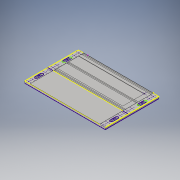
# Autodesk Inventor part: Fixture Base
Saved by Autodesk Inventor 2016 (Build 200138000, 138)
## iProperties
Created: 2016-04-07
Part Number: Fixture Base
Material: Generic
Document SubType Name: Modeling
Designer: Sam Clay
Density: 1 g/cm^3
Appearance: Default
Author: Sam Clay
Autodesk Inventor part; units mm, degrees
ref_plane "YZ Plane" through (0, 0, 0) normal (1, 0, 0) x (0, 1, 0)
ref_plane "XZ Plane" through (0, 0, 0) normal (0, 1, 0) x (-1, 0, 0)
ref_plane "XY Plane" through (0, 0, 0) normal (0, 0, 1) x (1, 0, 0)
sketch "Base Sketch" plane through (0, 0, 0) normal (0, 1, 0) x (-1, 0, 0)
  line L0 (0, 0) -> (660.4, 0)
  line L1 (660.4, 0) -> (660.4, 254)
  line L2 (660.4, 508) -> (0, 508)
  line L3 (0, 508) -> (0, 0)
  line L4 (0, 508) -> (-50.8, 508)
  line L5 (-50.8, 508) -> (-50.8, 254)
  line L6 (-50.8, 0) -> (0, 0)
  line L7 (0, 0) -> (0, 254)
  line L8 (660.4, 508) -> (711.2, 508)
  line L9 (711.2, 508) -> (711.2, 254)
  line L10 (711.2, 0) -> (660.4, 0)
  line L11 (660.4, 0) -> (660.4, 508)
  line L12 (711.2, 254) -> (-50.8, 254)
  line L13 (660.4, 254) -> (660.4, 508)
  line L14 (711.2, 254) -> (711.2, 0)
  line L15 (0, 254) -> (0, 508)
  line L16 (-50.8, 254) -> (-50.8, 0)
  dimension "d0" = 660.4
  dimension "d1" = 508
  dimension "d87" = 50.8
  dimension "d88" = 50.8
  dimension "d118" = 254
  constraints: 34 end point, 11 parallel, 8 perpendicular, 3 horizontal, 3 point on line
  measures "d0" distance of L2.end L2.start
  measures "d1" distance of L2.start L0.end
  measures "d87" distance of L6.end L6.start
  measures "d88" distance of L10.start L10.end
  measures "d118" distance between parallel lines of L0 L12
extrude "Base" add sketch "Base Sketch" along normal blind 19.05 contours L3 L12 L1 L0 | L3 L2 L11 L12
sketch "Tracks Sketch" plane through (0, 19.05, 0) normal (0, 1, 0) x (1, 0, 0)
  line L0 (0, 0) -> (-660.4, 0) projected
  line L1 (-660.4, 0) -> (-660.4, -508) projected
  line L2 (0, 0) -> (-660.4, 0)
  line L3 (-660.4, 0) -> (-660.4, -22.987)
  line L4 (-660.4, -22.987) -> (0, -22.987)
  line L5 (0, -22.987) -> (0, 0)
  line L6 (0, 0) -> (-38.1, 0)
  line L7 (-38.1, 0) -> (-38.1, -251.587)
  line L8 (-38.1, -251.587) -> (0, -251.587)
  line L9 (0, -251.587) -> (0, 0)
  line L10 (-38.1, -284.099) -> (-660.4, -284.099)
  line L11 (-660.4, -284.099) -> (-660.4, -264.287)
  line L12 (-660.4, -264.287) -> (-38.1, -264.287)
  line L13 (-38.1, -264.287) -> (-38.1, -284.099)
  line L14 (0, -48.387) -> (-660.4, -48.387)
  line L15 (-660.4, -48.387) -> (-660.4, -35.687)
  line L16 (-660.4, -35.687) -> (0, -35.687)
  line L17 (0, -35.687) -> (0, -48.387)
  line L18 (-38.1, -42.217) -> (-31.93, -48.387)
  line L19 (-38.1, -42.217) -> (-46.8257, -42.217) construction
  circle A0 centre (-40.4921, -50.7791) radius 8.89
  line L20 (-660.4, -3.175) -> (0, -3.175)
  line L21 (0, -508) -> (0, 0) projected
  line L22 (-38.1, -251.587) -> (-660.4, -251.587)
  line L23 (-660.4, -290.449) -> (0, -290.449)
  line L24 (-38.1, -284.099) -> (0, -284.099)
  line L25 (-38.1, -264.287) -> (0, -264.287)
  line L26 (-660.4, -309.499) -> (0, -309.499)
  line L27 (-660.4, -488.95) -> (0, -488.95)
  line L28 (-660.4, -508) -> (0, -508) projected
  line L29 (-44.45, -309.499) -> (-44.45, -488.95)
  line L30 (-615.95, -309.499) -> (-615.95, -488.95)
  line L31 (-660.4, -142.113) -> (0, -142.113)
  line L32 (-660.4, -161.925) -> (0, -161.925)
  line L33 (-660.4, -200.025) -> (0, -200.025)
  line L34 (-660.4, -219.837) -> (0, -219.837)
  line L35 (-660.4, -142.113) -> (-660.4, -161.925)
  line L36 (-660.4, -200.025) -> (-660.4, -219.837)
  line L37 (0, -200.025) -> (0, -219.837)
  line L38 (0, -142.113) -> (0, -161.925)
  point P0 (-38.1, -22.987)
  point P1 (-38.1, -48.387)
  point P2 (-38.1, -48.387)
  point P3 (-38.1, -3.175)
  dimension "d5" = 38.1
  dimension "d75" = 19.812
  dimension "d76" = 12.7
  dimension "d77" = 12.7
  dimension "d78" = 12.7
  dimension "d79" = 203.2
  dimension "d83" = 135
  dimension "d84" = 17.78
  dimension "d101" = 3.175
  dimension "d102" = 19.812
  dimension "d109" = 6.35
  dimension "d154" = 19.05
  dimension "d155" = 19.05
  dimension "d156" = 44.45
  dimension "d157" = 44.45
  dimension "d158" = 19.812
  dimension "d159" = 19.812
  dimension "d161" = 38.1
  dimension "d164" = 31.75
  constraints: 70 end point, 15 point on line, 13 horizontal, 9 perpendicular, 8 parallel, 4 coincident, 2 collinear, 2 point on circle, 2 vertical, 1 centre point, 1 equal length, 23 other
  measures "d5" distance of L8.end L7.end
  measures "d75" distance of L10.end L11.end
  measures "d76" distance from line of L8.end L12
  measures "d77" distance of L14.end L15.end
  measures "d78" distance between parallel lines of L4 L16
  measures "d79" distance from line of L14 L7.end
  measures "d83" angle of L19 L18
  measures "d84" diameter of A0
  measures "d101" distance between parallel lines of L0 L20
  measures "d102" distance between parallel lines of L4 L20
  measures "d109" distance between parallel lines of L23 L10
  measures "d154" distance between parallel lines of L23 L26
  measures "d155" distance between parallel lines of L28 L27
  measures "d157" distance of the line from the sketch origin of L29
  measures "d158" distance between parallel lines of L32 L31
  measures "d159" distance between parallel lines of L34 L33
  measures "d161" distance between parallel lines of L32 L33
  measures "d164" distance between parallel lines of L22 L34
extrude "Track Separator" cut sketch "Tracks Sketch" against normal blind 0.0254 contours L21 L23 L1 L10 L24
extrude "Pocket side" cut sketch "Tracks Sketch" against normal blind 3.175 contours L18 L14 L7 | A0 L18 | L7 L14 A0 | A0 L7 L14 | L14 A0 L7 L31 L1 | L7 A0 L14 | L7 L32 L1 L31 | L7 L33 L1 L32 | L7 L34 L1 L33 | L7 L22 L1 L34
extrude "Tracks" cut sketch "Tracks Sketch" against normal blind 9.8425 contours L5 L4 L7 L20 | L7 L4 L1 L20 | L21 L24 L13 L25 | L13 L10 L1 L12
extrude "Interior Tracks" cut sketch "Tracks Sketch" against normal blind 13.0175 contours L9 L32 L7 L31 | L7 L32 L1 L31
extrude "Lower Level" add sketch "Base Sketch" along normal blind 17.78 contours L6 L16 L12 L3 | L1 L12 L14 L10 | L12 L5 L4 L3 | L11 L8 L9 L12
sketch "Handle Sketch" plane through (0, 17.78, 0) normal (0, 1, 0) x (1, 0, 0)
  line L0 (-660.4, 0) -> (-711.2, 0) projected
  line L1 (-711.2, 0) -> (-711.2, -508) projected
  line L2 (50.8, -508) -> (50.8, 0) projected
  line L3 (-711.2, -508) -> (-660.4, -508) projected
  line L4 (25.4, -104.0628) -> (25.4, -162.6372) construction
  line L5 (12.7, -104.0628) -> (12.7, -162.6372)
  line L6 (38.1, -162.6372) -> (38.1, -104.0628)
  arc A0 (38.1, -104.0628) -> (12.7, -104.0628) centre (25.4, -104.0628) ccw
  arc A1 (12.7, -162.6372) -> (38.1, -162.6372) centre (25.4, -162.6372) ccw
  line L7 (-685.8, -103.8528) -> (-685.8, -162.8472) construction
  line L8 (-698.5, -103.8528) -> (-698.5, -162.8472)
  line L9 (-673.1, -162.8472) -> (-673.1, -103.8528)
  arc A2 (-673.1, -103.8528) -> (-698.5, -103.8528) centre (-685.8, -103.8528) ccw
  arc A3 (-698.5, -162.8472) -> (-673.1, -162.8472) centre (-685.8, -162.8472) ccw
  line L10 (0, -290.449) -> (-660.4, -290.449) projected
  line L11 (-660.4, -508) -> (0, -508) projected
  line L12 (50.8, 0) -> (0, 0) projected
  line L13 (-685.8, -423.799) -> (-685.8, -372.999) construction
  line L14 (-673.1, -423.799) -> (-673.1, -372.999)
  line L15 (-698.5, -372.999) -> (-698.5, -423.799)
  arc A4 (-698.5, -423.799) -> (-673.1, -423.799) centre (-685.8, -423.799) ccw
  arc A5 (-673.1, -372.999) -> (-698.5, -372.999) centre (-685.8, -372.999) ccw
  line L16 (25.4, -423.799) -> (25.4, -372.999) construction
  line L17 (38.1, -423.799) -> (38.1, -372.999)
  line L18 (12.7, -372.999) -> (12.7, -423.799)
  arc A6 (12.7, -423.799) -> (38.1, -423.799) centre (25.4, -423.799) ccw
  arc A7 (38.1, -372.999) -> (12.7, -372.999) centre (25.4, -372.999) ccw
  point P0 (-685.8, -25.4)
  point P1 (-685.8, -63.5)
  point P2 (-685.8, -457.2)
  point P3 (-622.3, 0)
  point P4 (25.4, -265.049)
  point P5 (25.4, -226.949)
  point P6 (25.4, -25.4)
  point P7 (-685.8, -495.3)
  point P8 (25.4, -63.5)
  point P9 (25.4, -133.35)
  point P10 (-685.8, -133.35)
  point P11 (-685.8, -226.949)
  point P12 (-685.8, -265.049)
  point P13 (-685.8, -303.149)
  point P14 (-685.8, -341.249)
  point P15 (25.4, -303.149)
  point P16 (25.4, -341.249)
  point P17 (25.4, -457.2)
  point P18 (25.4, -495.3)
  point P19 (-685.8, -398.399)
  point P20 (25.4, -398.399)
  dimension "d91" = 25.4
  dimension "d97" = 38.1
  dimension "d99" = 38.1
  dimension "d100" = 12.7
  dimension "d103" = 25.4
  dimension "d104" = 25.4
  dimension "d106" = 25.4
  dimension "d107" = 25.4
  dimension "d108" = 25.4
  dimension "d114" = 12.7
  dimension "d115" = 25.4
  dimension "d116" = 25.4
  dimension "d117" = 25.4
  dimension "d119" = 38.1
  dimension "d120" = 38.1
  dimension "d123" = 25.4
  dimension "d124" = 25.4
  dimension "d125" = 25.4
  dimension "d127" = 25.4
  dimension "d128" = 25.4
  dimension "d129" = 25.4
  dimension "d131" = 38.1
  dimension "d132" = 12.7
  dimension "d133" = 38.1
  dimension "d134" = 25.4
  dimension "d135" = 25.4
  dimension "d136" = 12.7
  dimension "d137" = 38.1
  dimension "d138" = 25.4
  dimension "d139" = 25.4
  dimension "d140" = 25.4
  dimension "d141" = 38.1
  dimension "d142" = 25.4
  dimension "d143" = 25.4
  dimension "d144" = 25.4
  dimension "d145" = 25.4
  dimension "d146" = 57.15
  dimension "d147" = 69.85
  dimension "d148" = 69.85
  dimension "d149" = 25.4
  dimension "d150" = 25.4
  dimension "d151" = 25.4
  dimension "d152" = 57.15
  dimension "d153" = 12.7
  constraints: 32 end point, 16 point on circle, 16 tangent, 8 centre point, 4 midpoint, 4 parallel, 4 vertical, 2 vertical alignment
  measures "d91" distance from line of point (-685.8, -25.4) L0
  measures "d97" distance of point (-685.8, -63.5) point (-685.8, -25.4)
  measures "d99" distance of point (-685.8, -457.2) point (-685.8, -495.3)
  measures "d100" distance from line of L3 point (-685.8, -495.3)
  measures "d103" distance from line of point (-685.8, -63.5) L1
  measures "d104" distance from line of L1 point (-685.8, -25.4)
  measures "d106" distance from line of L1 point (-685.8, -495.3)
  measures "d107" distance from line of L2 point (25.4, -25.4)
  measures "d108" distance from line of L2 point (25.4, -63.5)
  measures "d114" distance between parallel lines of L6 L4
  measures "d115" diameter of A3
  measures "d116" distance from line of L1 L7.start
  measures "d117" distance from line of L2 L4.start
  measures "d119" distance of point (-685.8, -265.049) point (-685.8, -226.949)
  measures "d120" distance of point (25.4, -226.949) point (25.4, -265.049)
  measures "d123" distance from line of L1 point (-685.8, -226.949)
  measures "d124" distance from line of L10 point (-685.8, -265.049)
  measures "d125" distance from line of L1 point (-685.8, -265.049)
  measures "d127" distance from line of L1 point (-685.8, -457.2)
  measures "d128" distance from line of L1 point (-685.8, -341.249)
  measures "d129" distance from line of L1 point (-685.8, -303.149)
  measures "d131" distance of point (-685.8, -303.149) point (-685.8, -341.249)
  measures "d132" distance from line of L10 point (25.4, -303.149)
  measures "d133" distance of point (25.4, -303.149) point (25.4, -341.249)
  measures "d134" distance from line of L2 point (25.4, -303.149)
  measures "d135" distance from line of L2 point (25.4, -341.249)
  measures "d136" distance from line of L11 point (25.4, -495.3)
  measures "d137" distance of point (25.4, -495.3) point (25.4, -457.2)
  measures "d138" distance from line of L2 point (25.4, -495.3)
  measures "d139" distance from line of L2 point (25.4, -457.2)
  measures "d140" distance from line of L12 point (25.4, -25.4)
  measures "d141" distance of point (25.4, -25.4) point (25.4, -63.5)
  measures "d142" distance from line of L10 point (25.4, -265.049)
  measures "d143" distance of point (-685.8, -398.399) L13.end
  measures "d144" diameter of A5
  measures "d145" distance from line of L1 point (-685.8, -398.399)
  measures "d146" distance of point (-685.8, -398.399) point (-685.8, -341.249)
  measures "d147" distance of point (-685.8, -63.5) point (-685.8, -133.35)
  measures "d148" distance of point (25.4, -63.5) point (25.4, -133.35)
  measures "d149" distance of point (25.4, -398.399) L16.end
  measures "d150" diameter of A7
  measures "d151" distance from line of L2 point (25.4, -398.399)
  measures "d152" distance of point (25.4, -341.249) point (25.4, -398.399)
  measures "d153" distance from line of point (-685.8, -303.149) L10
sketch "Origin Sketch" plane through (0, 19.05, 0) normal (0, 1, 0) x (1, 0, 0)
  line L0 (0, -290.449) -> (-660.4, -290.449) projected
  line L1 (-660.4, -290.449) -> (-711.2, -290.449)
  line L2 (-711.2, 0) -> (-711.2, -508) projected
  line L3 (0, -290.449) -> (50.8, -290.449)
  line L4 (50.8, -508) -> (50.8, 0) projected
  point P0 (0, 0)
  point P1 (-38.1, -48.387)
  point P2 (-38.1, -48.387)
  constraints: 4 end point, 3 point on line, 1 coincident, 1 horizontal
extrude "Handles" cut sketch "Handle Sketch" against normal through all
equation "\"d104\" = d103"
equation "\"d106\" = d103"
equation "\"d107\" = d103"
equation "\"d108\" = d103"
equation "\"d119\" = d97"
equation "\"d120\" = d97"
equation "\"d124\" = d91"
body "Solid1"
